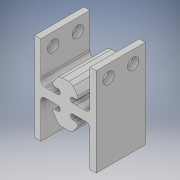
# Autodesk Inventor part: Actual
Saved by Autodesk Inventor 2018 (Build 220112000, 112)
## iProperties
Created: 2018-03-23
Part Number: Actual
Material: Generic
Document SubType Name: Modeling
Designer: Student
Density: 1 g/cm^3
Appearance: Default
Author: Student
Autodesk Inventor part; units mm, degrees
ref_plane "YZ Plane" through (0, 0, 0) normal (1, 0, 0) x (0, 1, 0)
ref_plane "XZ Plane" through (0, 0, 0) normal (0, 1, 0) x (-1, 0, 0)
sketch "Sketch3" plane through (0, 0, 0) normal (0, 0, 1) x (1, 0, 0)
  line L0 (-4.6029, -3.7799) -> (-2.2865, -0.551)
  arc A0 (0.0488, 0.3695) -> (-2.2865, -0.551) centre (-0.0488, -2.8055) ccw
  line L1 (-1.8769, -5.6171) -> (-3.8542, -5.6171)
  line L2 (-2.9065, -8.1571) -> (-1.8769, -8.1571)
  line L3 (-7.8411, -8.2042) -> (-3.9225, -8.1571)
  line L4 (-2.9065, -8.1571) -> (-3.9225, -8.1571)
  line L5 (1.7093, 4.4958) -> (1.7093, -14.4322)
  line L6 (-8.8571, -8.204) -> (-7.8411, -8.2042)
  arc A1 (-10.9906, -6.0706) -> (-8.8571, -8.204) centre (-8.8825, -6.096) ccw
  arc A2 (-10.9906, -6.0706) -> (-8.8571, -8.204) centre (-8.8825, -6.096) ccw
  line L7 (-10.9907, -5.0546) -> (-10.9906, -6.0706)
  line L8 (-10.9907, 12.258) -> (-10.9907, -5.0546)
  line L9 (-10.9907, -5.0546) -> (-10.9907, 12.258)
  line L10 (-11.2451, -10.6176) -> (1.7093, -10.6176)
  arc A3 (-10.9907, 12.258) -> (-10.9907, 12.258) centre (-10.9907, 11.75) ccw
  line L11 (-14.1657, 12.258) -> (-10.9907, 12.258)
  line L12 (-11.2451, -10.6176) -> (-14.1657, -10.6176)
  line L13 (-14.1657, 12.258) -> (-14.1657, -10.6176)
  arc A4 (-4.6029, -3.7799) -> (-3.8542, -5.6171) centre (-3.5384, -4.4173) ccw
  arc A5 (-1.8769, -8.1571) -> (-1.8769, -5.6171) centre (-2.2619, -6.8871) ccw
  line L14 (0.0488, 0.3695) -> (1.7093, 0.3695)
  line L15 (8.0214, -3.7799) -> (5.705, -0.551)
  arc A6 (5.705, -0.551) -> (3.3697, 0.3695) centre (3.4673, -2.8055) ccw
  line L16 (5.2954, -5.6171) -> (7.2727, -5.6171)
  line L17 (6.325, -8.1571) -> (5.2954, -8.1571)
  line L18 (11.2597, -8.2042) -> (7.341, -8.1571)
  line L19 (6.325, -8.1571) -> (7.341, -8.1571)
  line L20 (12.2757, -8.204) -> (11.2597, -8.2042)
  arc A7 (12.2757, -8.204) -> (14.4091, -6.0706) centre (12.3011, -6.096) ccw
  arc A8 (12.2757, -8.204) -> (14.4091, -6.0706) centre (12.3011, -6.096) ccw
  line L21 (14.4093, -5.0546) -> (14.4091, -6.0706)
  line L22 (14.4093, 12.258) -> (14.4093, -5.0546)
  line L23 (14.4093, -5.0546) -> (14.4093, 12.258)
  line L24 (14.6636, -10.6176) -> (1.7093, -10.6176)
  arc A9 (14.4093, 12.258) -> (14.4093, 12.258) centre (14.4093, 11.75) ccw
  line L25 (17.5843, 12.258) -> (14.4093, 12.258)
  line L26 (14.6636, -10.6176) -> (17.5843, -10.6176)
  line L27 (17.5843, 12.258) -> (17.5843, -10.6176)
  arc A10 (7.2727, -5.6171) -> (8.0214, -3.7799) centre (6.9569, -4.4173) ccw
  arc A11 (5.2954, -5.6171) -> (5.2954, -8.1571) centre (5.6804, -6.8871) ccw
  line L28 (3.3697, 0.3695) -> (1.7093, 0.3695)
  point P0 (0, 0)
  point P1 (3.4185, 0)
  point P2 (1.7093, -6.8871)
  point P3 (4.3533, -6.8871)
  dimension "d8" = 3.175
  dimension "d34" = 2.54
  dimension "d37" = 11.1268
  dimension "d38" = 7.2566
  constraints: 58 end point, 25 point on circle, 24 symmetric about line, 12 centre point, 5 point on line, 2 coincident, 2 horizontal, 2 perpendicular, 2 vertical, 1 horizontal alignment, 6 other
  measures "d8" distance of L11.start L9.end
  measures "d34" distance between parallel lines of L4 L1
  measures "d37" distance of L16.end L1.end
  measures "d38" distance from line of L28 point (1.709, -6.887)
extrude "Extrusion8" add sketch "Sketch3" along normal blind 25.4 contours L0 A0 L14 L5 L10 L12 L13 L11 A3 L8 L7 A1 L6 L3 L4 L2 A5 L1 A4 | L28 A6 L15 A10 L16 A11 L17 L19 L18 L20 A7 L21 L22 A9 L25 L27 L26 L24 L5 | L8 A3 | A9 L22 picked at (-11.1588, 11.7704) picked at (14.5744, 11.7123)
ref_plane "Work Plane1" through (212.0306, -10.6176, 0) normal (-0.006, -1, 0) x (0, 0, -1)
mirror "Mirror2" about plane through (1.7093, -10.6176, 0) normal (0, -1, 0) of "Extrusion8"
sketch "Sketch12" plane through (17.5843, 12.258, 25.4) normal (1, 0, 0) x (0, 0, -1)
  line L0 (25.4, 0) -> (25.4, -45.7513) projected
  line L1 (25.4, 0) -> (0, 0) projected
  line L2 (0, 0) -> (0, -45.7513) projected
  line L3 (25.4, -45.7513) -> (0, -45.7513) projected
  line L4 (0, 0) -> (6.35, 0) construction
  line L5 (25.4, 0) -> (0, 0) construction
  line L6 (0, 0) -> (0, -6.35) construction
  line L7 (0, -17.3126) -> (0, 0) construction
  circle A0 centre (6.35, -6.35) radius 2.921
  line L8 (12.7, 0) -> (12.7, -45.7513)
  line L9 (25.4, -45.7513) -> (0, -45.7513) projected
  circle A1 centre (19.05, -6.35) radius 2.921
  point P0 (25.4, -12.258)
  dimension "d42" = 6.35
  dimension "d43" = 6.35
  dimension "d44" = 5.842
  constraints: 6 end point, 2 centre point, 2 midpoint, 2 point on line, 1 horizontal alignment, 1 symmetric about line, 1 vertical alignment, 1 other
  measures "d42" distance of L1.end L4.end
  measures "d43" distance of L1.end L6.end
  measures "d44" diameter of A0
extrude "Extrusion9" cut sketch "Sketch12" against normal through all contours A0 | A1
body "Solid2"
